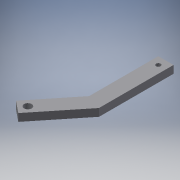
# Autodesk Inventor part: bras
Saved by Autodesk Inventor 2017 SP1 (Build 210196100, 196)
## iProperties
Part Number: bras
Material: Générique
Document SubType Name: Modeling
Designer: Biscuit
Density: 1 g/cm^3
Appearance: Par défaut
Author: Biscuit
Autodesk Inventor part; units mm, degrees
ref_plane "YZ Plane" through (0, 0, 0) normal (1, 0, 0) x (0, 1, 0)
ref_plane "XZ Plane" through (0, 0, 0) normal (0, 1, 0) x (-1, 0, 0)
ref_plane "XY Plane" through (0, 0, 0) normal (0, 0, 1) x (1, 0, 0)
sketch "Esquisse1" plane through (0, 0, 0) normal (0, 0, 1) x (1, 0, 0)
  line L0 (0, 0) -> (13.4419, 0)
  line L1 (13.4419, 0) -> (13.4419, -32.6795)
  line L2 (13.4419, -32.6795) -> (-12.1883, -77.0723)
  line L3 (-12.1883, -77.0723) -> (-20.8486, -72.0723)
  line L4 (-20.8486, -72.0723) -> (3.4419, -30)
  line L5 (3.4419, -30) -> (3.4419, 0)
  line L6 (3.4419, 0) -> (13.4419, 0)
  circle A0 centre (8.4419, -5) radius 1.5
  circle A1 centre (-14.0184, -70.2421) radius 2.5
  dimension "d0" = 5
  dimension "d1" = 5
  dimension "d2" = 10
  dimension "d3" = 5
  dimension "d4" = 5
  dimension "d5" = 5
  dimension "d6" = 3
  dimension "d7" = 65
  dimension "d9" = 150
  dimension "d13" = 25
  constraints: 14 end point, 3 perpendicular, 2 centre point, 1 collinear, 1 equal length, 1 horizontal, 1 parallel, 1 point on line
  measures "d0" distance from line of L2 A1.centre
  measures "d1" distance from line of L3 A1.centre
  measures "d2" distance of L5.end L0.end
  measures "d3" diameter of A1
  measures "d4" distance from line of L1 A0.centre
  measures "d5" distance from line of L0 A0.centre
  measures "d6" diameter of A0
  measures "d9" angle of L4 L5
  measures "d13" vertical distance of L4.end A0.centre
extrude "Extrusion1" add sketch "Esquisse1" along normal blind 5
fillet "Congé1" radius 5 4 edges at (-20.8486, -72.0723, 2.5) (-12.1883, -77.0723, 2.5) (13.4419, 0, 2.5) (3.4419, 0, 2.5)
